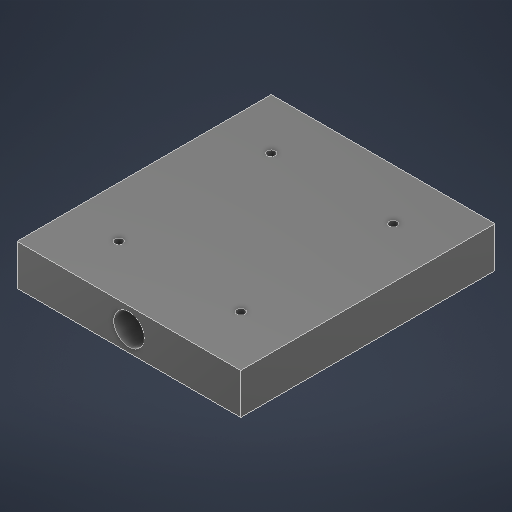
# Autodesk Inventor part: SACMI DPA TILES GRIP FIXED SUPPORT
Saved by Autodesk Inventor 2025 (Build 290162000, 162)
## iProperties
Created: 2024-05-27
Part Number: SACMI DPA TILES GRIP FIXED SUPPORT
Material: Generic
Document SubType Name: Modeling
Designer: zulet
Density: 1 g/cm^3
Appearance: Smooth - Black
Author: zulet
Autodesk Inventor part; units mm, degrees
ref_plane "YZ Plane" through (0, 0, 0) normal (1, 0, 0) x (0, 1, 0)
ref_plane "XZ Plane" through (0, 0, 0) normal (0, 1, 0) x (-1, 0, 0)
ref_plane "XY Plane" through (0, 0, 0) normal (0, 0, 1) x (1, 0, 0)
sketch "Sketch1" plane through (0, 0, 0) normal (0, 1, 0) x (-1, 0, 0)
  line L0 (110, -125) -> (-110, -125)
  line L1 (-110, -125) -> (-110, 125)
  line L2 (-110, 125) -> (110, 125)
  line L3 (110, 125) -> (110, -125)
  line L4 (110, -125) -> (-110, 125) construction
  line L5 (-110, -125) -> (110, 125) construction
  line L6 (-60, 75) -> (60, 75) construction
  line L7 (60, 75) -> (60, -75) construction
  line L8 (60, -75) -> (-60, -75) construction
  line L9 (-60, -75) -> (-60, 75) construction
  line L10 (-60, 75) -> (60, -75) construction
  line L11 (60, 75) -> (-60, -75) construction
  point P0 (0, 0)
  dimension "d0" = 220
  dimension "d1" = 250
  dimension "d2" = 120
  dimension "d3" = 150
  constraints: 24 end point, 4 coincident, 4 midpoint, 4 parallel, 2 horizontal, 2 perpendicular
  measures "d0" distance of L1.end L2.end
  measures "d1" distance of L0.end L1.end
  measures "d2" distance of L7.end L8.end
  measures "d3" distance of L6.end L7.end
extrude "Extrusion1" add sketch "Sketch1" along normal blind 40
hole "Hole1" at (-60, 0, -75) at (60, 0, -75) at (60, 0, 75) at (-60, 0, 75) direction (0, 1, 0) diameter 8 end through all
sketch "Sketch2" plane through (-110, 0, 125) normal (0, 0, 1) x (1, 0, 0)
  line L0 (0, 0) -> (220, 0) construction
  line L1 (0, 40) -> (220, 40) construction
  line L2 (220, 0) -> (0, 40) construction
  line L3 (0, 0) -> (220, 40) construction
  circle A0 centre (110, 20) radius 15
  point P0 (110, 0)
  dimension "d13" = 30
  constraints: 4 end point, 1 centre point, 1 midpoint
  measures "d13" diameter of A0
extrude "Extrusion2" cut sketch "Sketch2" against normal through all
body "Solid1"
